Autodesk Fusion 360 part; units mm, degrees
note: some values were not read from the file. Set by a fixed rule: which sketch regions a step uses.
(part 2 of 2)
sketch "Sketch10" plane through (0, 25.4, 0) normal (0, 1, 0) x (-1, 0, 0)
  line L0 (-83.2873, -65.9474) -> (-83.2873, -59.1973)
  line L1 (-83.2873, -59.1973) -> (-104.0797, -59.1973)
  arc A0 (-123.262, -24.2329) -> (-104.0797, -59.1973) centre (-37.6354, -0.0001) ccw
  line L2 (-123.262, -24.2329) -> (-104.2867, -24.2329)
  line L3 (-104.2867, -24.2329) -> (-24.2324, -24.2327)
  line L4 (-24.2324, -24.2327) -> (-24.2324, -59.1973)
  line L5 (-24.2324, -59.1973) -> (-24.3061, -59.1973)
  line L6 (-24.3061, -59.1973) -> (-79.2873, -59.1973)
  line L7 (-79.2873, -59.1973) -> (-79.2873, -65.9474)
  line L8 (-79.2873, -65.9474) -> (-65.947, -65.9474)
  line L9 (-65.947, -65.9474) -> (-65.947, -107.6618)
  line L10 (-65.947, -107.6618) -> (-62.572, -107.6618)
  line L11 (-62.572, -107.6618) -> (-59.197, -107.6619)
  line L12 (-59.197, -107.6619) -> (-59.197, -107.6618)
  line L13 (-59.197, -107.6618) -> (65.9471, -107.6618)
  line L14 (65.9471, -107.6618) -> (65.9472, -104.2868)
  line L15 (65.9472, -104.2868) -> (65.9471, -65.9472)
  line L16 (65.9471, -65.9472) -> (100.9118, -65.9471)
  line L17 (100.9118, -65.9471) -> (100.9118, -104.2868)
  line L18 (100.9118, -104.2868) -> (107.6618, -104.2868)
  line L19 (107.6618, -104.2868) -> (107.6618, -23.7396)
  arc A1 (107.6618, -23.7396) -> (107.6618, 23.7395) centre (102.4721, -0.0001) ccw
  line L20 (107.6618, 23.7395) -> (100.9118, 23.7395)
  line L21 (100.9118, 23.7395) -> (100.9118, 17.4823)
  line L22 (100.9118, 17.4823) -> (104.2868, 17.4823)
  arc A2 (104.2868, -17.4824) -> (104.2868, 17.4823) centre (102.443, -0.0001) ccw
  line L23 (104.2868, -17.4824) -> (100.9118, -17.4824)
  line L24 (100.9118, -17.4824) -> (100.9118, -59.1971)
  line L25 (100.9118, -59.1971) -> (65.9471, -59.1972)
  line L26 (65.9471, -59.1972) -> (65.947, -17.4824)
  line L27 (65.947, -17.4824) -> (-17.4824, -17.4824)
  line L28 (-17.4824, -17.4824) -> (-17.4824, 17.4823)
  line L29 (-17.4824, 17.4823) -> (17.7085, 17.4823)
  arc A3 (17.7085, 17.4823) -> (65.7207, 17.4823) centre (41.7146, 20.7869) ccw
  line L30 (65.7207, 17.4823) -> (96.9118, 17.4823)
  line L31 (96.9118, 17.4823) -> (96.9118, 24.2323)
  line L32 (96.9118, 24.2323) -> (62.5606, 24.2322)
  line L33 (62.5606, 24.2322) -> (59.1856, 24.2322)
  line L34 (59.1856, 24.2322) -> (59.197, 20.8573)
  arc A4 (24.2323, 20.8573) -> (59.197, 20.8573) centre (41.7146, 20.7869) ccw
  line L35 (24.2323, 20.8573) -> (24.2323, 24.2322)
  line L36 (24.2323, 24.2322) -> (20.8573, 24.2323)
  line L37 (20.8573, 24.2323) -> (-17.4824, 24.2323)
  line L38 (-17.4824, 24.2323) -> (-17.4825, 100.9119)
  line L39 (-17.4825, 100.9119) -> (17.4821, 100.912)
  line L40 (17.4821, 100.912) -> (17.4821, 59.197)
  line L41 (17.4821, 59.197) -> (20.8571, 59.197)
  line L42 (20.8571, 59.197) -> (65.9469, 59.197)
  line L43 (65.9469, 59.197) -> (65.9469, 62.572)
  line L44 (65.9469, 62.572) -> (65.9468, 100.9119)
  line L45 (65.9468, 100.9119) -> (100.9118, 100.9119)
  line L46 (100.9118, 100.9119) -> (100.9118, 27.7395)
  line L47 (100.9118, 27.7395) -> (107.6618, 27.7395)
  line L48 (107.6618, 27.7395) -> (107.6618, 104.287)
  line L49 (107.6618, 104.287) -> (104.2868, 107.6568)
  line L50 (104.2868, 107.6568) -> (63.9876, 107.6568)
  arc A5 (63.9876, 107.6568) -> (-65.9473, 104.2867) centre (-0.0002, 68.2001) ccw
  line L51 (-65.9473, 104.2867) -> (-65.9473, 65.947)
  line L52 (-65.9473, 65.947) -> (-104.2867, 65.947)
  arc A6 (-104.2867, 65.947) -> (-107.6617, -63.1217) centre (-42.5552, -0.2457) ccw
  line L53 (-107.6617, -63.1217) -> (-107.6617, -104.2871)
  line L54 (-107.6617, -104.2871) -> (-104.2867, -104.2868)
  line L55 (-104.2867, -104.2868) -> (-100.9117, -104.287)
  line L56 (-100.9117, -104.287) -> (-100.9117, -65.9474)
  line L57 (-100.9117, -65.9474) -> (-83.2873, -65.9474)
  line L58 (-17.4824, -59.1973) -> (-17.4824, -24.2327)
  line L59 (-17.4824, -24.2327) -> (59.1971, -24.2325)
  line L60 (59.1971, -24.2325) -> (59.1971, -59.1972)
  line L61 (59.1971, -59.1972) -> (20.8574, -59.1972)
  line L62 (20.8574, -59.1972) -> (-17.4824, -59.1973)
  line L63 (-17.4824, -65.9474) -> (17.4824, -65.9473)
  line L64 (17.4824, -65.9473) -> (17.4824, -100.9118)
  line L65 (17.4824, -100.9118) -> (-59.197, -100.9118)
  line L66 (-59.197, -100.9118) -> (-59.197, -65.9474)
  line L67 (-59.197, -65.9474) -> (-17.4824, -65.9474)
  line L68 (-17.4824, -65.9474) -> (-17.4824, -65.9474)
  line L69 (24.2322, 104.287) -> (24.2321, 107.662)
  line L70 (24.2321, 107.662) -> (-56.8908, 107.6591)
  arc A7 (59.1968, 104.2869) -> (-56.8908, 107.6591) centre (-0.0002, 66.274) ccw
  line L71 (59.1968, 104.2869) -> (59.1969, 65.947)
  line L72 (59.1969, 65.947) -> (24.2322, 65.9469)
  line L73 (24.2322, 65.9469) -> (24.2322, 104.287)
  line L74 (24.2324, -100.9118) -> (24.2324, -65.9473)
  line L75 (24.2324, -65.9473) -> (59.1971, -65.9472)
  line L76 (59.1971, -65.9472) -> (59.1971, -100.9118)
  line L77 (59.1971, -100.9118) -> (24.2324, -100.9118)
  line L78 (-24.2324, 17.4823) -> (-24.2324, -17.4824)
  line L79 (-24.2324, -17.4824) -> (-100.9117, -17.4824)
  line L80 (-100.9117, -17.4824) -> (-100.9117, 17.4823)
  line L81 (-100.9117, 17.4823) -> (-24.2324, 17.4823)
  line L82 (-59.1972, 59.197) -> (-59.1973, 100.9118)
  line L83 (-59.1973, 100.9118) -> (-24.2324, 100.9119)
  line L84 (-24.2324, 100.9119) -> (-24.2324, 24.2323)
  line L85 (-24.2324, 24.2323) -> (-107.6617, 24.2323)
  line L86 (-107.6617, 24.2323) -> (-107.6616, -17.4824)
  line L87 (-107.6616, -17.4824) -> (-124.8909, -17.4824)
  arc A8 (-104.0798, 59.197) -> (-124.8909, -17.4824) centre (-37.6354, -0.0001) ccw
  line L88 (-104.0798, 59.197) -> (-59.1972, 59.197)
  line L89 (-17.4824, -59.1973) -> (-24.2324, -59.1973)
  line L90 (-24.2324, -59.1973) -> (-24.2324, -65.9474)
  line L91 (-24.2324, -65.9474) -> (-17.4824, -65.9474)
  line L92 (-17.4824, -65.9474) -> (-17.4824, -59.1973)
  dimension "d79" = 6.75
  measures "d79" distance of L58.start L4.end
extrude "Extrude11" add sketch "Sketch10" along normal blind 7 contours L67 L89 L90 L91 L92 bodies 2 1
sketch "Sketch11" plane through (0, 25.4, 0) normal (0, 1, 0) x (-1, 0, 0)
  line L0 (-24.2324, -65.9474) -> (-24.2324, -59.1973)
  line L1 (-24.2324, -59.1973) -> (-24.3061, -59.1973)
  line L2 (-24.3061, -59.1973) -> (-79.2873, -59.1973)
  line L3 (-79.2873, -59.1973) -> (-79.2873, -65.9474)
  line L4 (-79.2873, -65.9474) -> (-65.947, -65.9474)
  line L5 (-65.947, -65.9474) -> (-65.947, -107.6618)
  line L6 (-65.947, -107.6618) -> (-62.572, -107.6618)
  line L7 (-62.572, -107.6618) -> (-59.197, -107.6619)
  line L8 (-59.197, -107.6619) -> (-59.197, -107.6618)
  line L9 (-59.197, -107.6618) -> (65.9471, -107.6618)
  line L10 (65.9471, -107.6618) -> (65.9472, -104.2868)
  line L11 (65.9472, -104.2868) -> (65.9471, -65.9472)
  line L12 (65.9471, -65.9472) -> (100.9118, -65.9471)
  line L13 (100.9118, -65.9471) -> (100.9118, -104.2868)
  line L14 (100.9118, -104.2868) -> (107.6618, -104.2868)
  line L15 (107.6618, -104.2868) -> (107.6618, -23.7396)
  arc A0 (107.6618, -23.7396) -> (107.6618, 23.7395) centre (102.4721, -0.0001) ccw
  line L16 (107.6618, 23.7395) -> (100.9118, 23.7395)
  line L17 (100.9118, 23.7395) -> (100.9118, 17.4823)
  line L18 (100.9118, 17.4823) -> (104.2868, 17.4823)
  arc A1 (104.2868, -17.4824) -> (104.2868, 17.4823) centre (102.443, -0.0001) ccw
  line L19 (104.2868, -17.4824) -> (100.9118, -17.4824)
  line L20 (100.9118, -17.4824) -> (100.9118, -59.1971)
  line L21 (100.9118, -59.1971) -> (65.9471, -59.1972)
  line L22 (65.9471, -59.1972) -> (65.947, -17.4824)
  line L23 (65.947, -17.4824) -> (-17.4824, -17.4824)
  line L24 (-17.4824, -17.4824) -> (-17.4824, 17.4823)
  line L25 (-17.4824, 17.4823) -> (17.7085, 17.4823)
  arc A2 (17.7085, 17.4823) -> (65.7207, 17.4823) centre (41.7146, 20.7869) ccw
  line L26 (65.7207, 17.4823) -> (96.9118, 17.4823)
  line L27 (96.9118, 17.4823) -> (96.9118, 24.2323)
  line L28 (96.9118, 24.2323) -> (62.5606, 24.2322)
  line L29 (62.5606, 24.2322) -> (59.1856, 24.2322)
  line L30 (59.1856, 24.2322) -> (59.197, 20.8573)
  arc A3 (24.2323, 20.8573) -> (59.197, 20.8573) centre (41.7146, 20.7869) ccw
  line L31 (24.2323, 20.8573) -> (24.2323, 24.2322)
  line L32 (24.2323, 24.2322) -> (20.8573, 24.2323)
  line L33 (20.8573, 24.2323) -> (-17.4824, 24.2323)
  line L34 (-17.4824, 24.2323) -> (-17.4825, 100.9119)
  line L35 (-17.4825, 100.9119) -> (17.4821, 100.912)
  line L36 (17.4821, 100.912) -> (17.4821, 59.197)
  line L37 (17.4821, 59.197) -> (20.8571, 59.197)
  line L38 (20.8571, 59.197) -> (65.9469, 59.197)
  line L39 (65.9469, 59.197) -> (65.9469, 62.572)
  line L40 (65.9469, 62.572) -> (65.9468, 100.9119)
  line L41 (65.9468, 100.9119) -> (100.9118, 100.9119)
  line L42 (100.9118, 100.9119) -> (100.9118, 27.7395)
  line L43 (100.9118, 27.7395) -> (107.6618, 27.7395)
  line L44 (107.6618, 27.7395) -> (107.6618, 104.287)
  line L45 (107.6618, 104.287) -> (104.2868, 107.6568)
  line L46 (104.2868, 107.6568) -> (63.9876, 107.6568)
  arc A4 (63.9876, 107.6568) -> (-65.9473, 104.2867) centre (-0.0002, 68.2001) ccw
  line L47 (-65.9473, 104.2867) -> (-65.9473, 65.947)
  line L48 (-65.9473, 65.947) -> (-104.2867, 65.947)
  arc A5 (-104.2867, 65.947) -> (-107.6617, -63.1217) centre (-42.5552, -0.2457) ccw
  line L49 (-107.6617, -63.1217) -> (-107.6617, -104.2871)
  line L50 (-107.6617, -104.2871) -> (-104.2867, -104.2868)
  line L51 (-104.2867, -104.2868) -> (-100.9117, -104.287)
  line L52 (-100.9117, -104.287) -> (-100.9117, -65.9474)
  line L53 (-100.9117, -65.9474) -> (-83.2873, -65.9474)
  line L54 (-83.2873, -65.9474) -> (-83.2873, -59.1973)
  line L55 (-83.2873, -59.1973) -> (-104.0797, -59.1973)
  arc A6 (-123.262, -24.2329) -> (-104.0797, -59.1973) centre (-37.6354, -0.0001) ccw
  line L56 (-123.262, -24.2329) -> (-104.2867, -24.2329)
  line L57 (-104.2867, -24.2329) -> (-24.2324, -24.2327)
  line L58 (-24.2324, -24.2327) -> (-24.2324, -59.1973)
  line L59 (-24.2324, -59.1973) -> (-17.4824, -59.1973)
  line L60 (-17.4824, -59.1973) -> (-17.4824, -24.2327)
  line L61 (-17.4824, -24.2327) -> (59.1971, -24.2325)
  line L62 (59.1971, -24.2325) -> (59.1971, -59.1972)
  line L63 (59.1971, -59.1972) -> (20.8574, -59.1972)
  line L64 (20.8574, -59.1972) -> (-17.4824, -59.1973)
  line L65 (-17.4824, -59.1973) -> (-17.4824, -65.9474)
  line L66 (-17.4824, -65.9474) -> (17.4824, -65.9473)
  line L67 (17.4824, -65.9473) -> (17.4824, -100.9118)
  line L68 (17.4824, -100.9118) -> (-59.197, -100.9118)
  line L69 (-59.197, -100.9118) -> (-59.197, -65.9474)
  line L70 (-59.197, -65.9474) -> (-24.2324, -65.9474)
  line L71 (24.2322, 104.287) -> (24.2321, 107.662)
  line L72 (24.2321, 107.662) -> (-56.8908, 107.6591)
  arc A7 (59.1968, 104.2869) -> (-56.8908, 107.6591) centre (-0.0002, 66.274) ccw
  line L73 (59.1968, 104.2869) -> (59.1969, 65.947)
  line L74 (59.1969, 65.947) -> (24.2322, 65.9469)
  line L75 (24.2322, 65.9469) -> (24.2322, 104.287)
  line L76 (24.2324, -100.9118) -> (24.2324, -65.9473)
  line L77 (24.2324, -65.9473) -> (59.1971, -65.9472)
  line L78 (59.1971, -65.9472) -> (59.1971, -100.9118)
  line L79 (59.1971, -100.9118) -> (24.2324, -100.9118)
  line L80 (-24.2324, 17.4823) -> (-24.2324, -17.4824)
  line L81 (-24.2324, -17.4824) -> (-100.9117, -17.4824)
  line L82 (-100.9117, -17.4824) -> (-100.9117, 17.4823)
  line L83 (-100.9117, 17.4823) -> (-24.2324, 17.4823)
  line L84 (-59.1972, 59.197) -> (-59.1973, 100.9118)
  line L85 (-59.1973, 100.9118) -> (-24.2324, 100.9119)
  line L86 (-24.2324, 100.9119) -> (-24.2324, 24.2323)
  line L87 (-24.2324, 24.2323) -> (-107.6617, 24.2323)
  line L88 (-107.6617, 24.2323) -> (-107.6616, -17.4824)
  line L89 (-107.6616, -17.4824) -> (-124.8909, -17.4824)
  arc A8 (-104.0798, 59.197) -> (-124.8909, -17.4824) centre (-37.6354, -0.0001) ccw
  line L90 (-104.0798, 59.197) -> (-59.1972, 59.197)
  line L91 (-100.9117, -2.7929) -> (-107.6616, -2.7929)
  line L92 (-107.6616, -2.7929) -> (-107.6616, 1.2071)
  line L93 (-107.6616, 1.2071) -> (-100.9117, 1.2071)
  line L94 (-100.9117, 1.2071) -> (-100.9117, -2.7929)
  dimension "d82" = 4
  measures "d82" distance of L91.start L93.end
extrude "Extrude12" add sketch "Sketch11" along normal blind 7 separate body contours L82 L88 L91 L92 L93 L94 makes body 3
sketch "Sketch12" plane through (0, 25.4, 0) normal (0, 1, 0) x (-1, 0, 0)
  line L0 (-24.2324, -65.9474) -> (-24.2324, -59.1973)
  line L1 (-24.2324, -59.1973) -> (-24.3061, -59.1973)
  line L2 (-24.3061, -59.1973) -> (-79.2873, -59.1973)
  line L3 (-79.2873, -59.1973) -> (-79.2873, -65.9474)
  line L4 (-79.2873, -65.9474) -> (-65.947, -65.9474)
  line L5 (-65.947, -65.9474) -> (-65.947, -107.6618)
  line L6 (-65.947, -107.6618) -> (-62.572, -107.6618)
  line L7 (-62.572, -107.6618) -> (-59.197, -107.6619)
  line L8 (-59.197, -107.6619) -> (-59.197, -107.6618)
  line L9 (-59.197, -107.6618) -> (65.9471, -107.6618)
  line L10 (65.9471, -107.6618) -> (65.9472, -104.2868)
  line L11 (65.9472, -104.2868) -> (65.9471, -65.9472)
  line L12 (65.9471, -65.9472) -> (100.9118, -65.9471)
  line L13 (100.9118, -65.9471) -> (100.9118, -104.2868)
  line L14 (100.9118, -104.2868) -> (107.6618, -104.2868)
  line L15 (107.6618, -104.2868) -> (107.6618, -23.7396)
  arc A0 (107.6618, -23.7396) -> (107.6618, 23.7395) centre (102.4721, -0.0001) ccw
  line L16 (107.6618, 23.7395) -> (100.9118, 23.7395)
  line L17 (100.9118, 23.7395) -> (100.9118, 17.4823)
  line L18 (100.9118, 17.4823) -> (104.2868, 17.4823)
  arc A1 (104.2868, -17.4824) -> (104.2868, 17.4823) centre (102.443, -0.0001) ccw
  line L19 (104.2868, -17.4824) -> (100.9118, -17.4824)
  line L20 (100.9118, -17.4824) -> (100.9118, -59.1971)
  line L21 (100.9118, -59.1971) -> (65.9471, -59.1972)
  line L22 (65.9471, -59.1972) -> (65.947, -17.4824)
  line L23 (65.947, -17.4824) -> (-17.4824, -17.4824)
  line L24 (-17.4824, -17.4824) -> (-17.4824, 17.4823)
  line L25 (-17.4824, 17.4823) -> (17.7085, 17.4823)
  arc A2 (17.7085, 17.4823) -> (65.7207, 17.4823) centre (41.7146, 20.7869) ccw
  line L26 (65.7207, 17.4823) -> (96.9118, 17.4823)
  line L27 (96.9118, 17.4823) -> (96.9118, 24.2323)
  line L28 (96.9118, 24.2323) -> (62.5606, 24.2322)
  line L29 (62.5606, 24.2322) -> (59.1856, 24.2322)
  line L30 (59.1856, 24.2322) -> (59.197, 20.8573)
  arc A3 (24.2323, 20.8573) -> (59.197, 20.8573) centre (41.7146, 20.7869) ccw
  line L31 (24.2323, 20.8573) -> (24.2323, 24.2322)
  line L32 (24.2323, 24.2322) -> (20.8573, 24.2323)
  line L33 (20.8573, 24.2323) -> (-17.4824, 24.2323)
  line L34 (-17.4824, 24.2323) -> (-17.4825, 100.9119)
  line L35 (-17.4825, 100.9119) -> (17.4821, 100.912)
  line L36 (17.4821, 100.912) -> (17.4821, 59.197)
  line L37 (17.4821, 59.197) -> (20.8571, 59.197)
  line L38 (20.8571, 59.197) -> (65.9469, 59.197)
  line L39 (65.9469, 59.197) -> (65.9469, 62.572)
  line L40 (65.9469, 62.572) -> (65.9468, 100.9119)
  line L41 (65.9468, 100.9119) -> (100.9118, 100.9119)
  line L42 (100.9118, 100.9119) -> (100.9118, 27.7395)
  line L43 (100.9118, 27.7395) -> (107.6618, 27.7395)
  line L44 (107.6618, 27.7395) -> (107.6618, 104.287)
  line L45 (107.6618, 104.287) -> (104.2868, 107.6568)
  line L46 (104.2868, 107.6568) -> (63.9876, 107.6568)
  arc A4 (63.9876, 107.6568) -> (-65.9473, 104.2867) centre (-0.0002, 68.2001) ccw
  line L47 (-65.9473, 104.2867) -> (-65.9473, 65.947)
  line L48 (-65.9473, 65.947) -> (-104.2867, 65.947)
  arc A5 (-104.2867, 65.947) -> (-107.6617, -63.1217) centre (-42.5552, -0.2457) ccw
  line L49 (-107.6617, -63.1217) -> (-107.6617, -104.2871)
  line L50 (-107.6617, -104.2871) -> (-104.2867, -104.2868)
  line L51 (-104.2867, -104.2868) -> (-100.9117, -104.287)
  line L52 (-100.9117, -104.287) -> (-100.9117, -65.9474)
  line L53 (-100.9117, -65.9474) -> (-83.2873, -65.9474)
  line L54 (-83.2873, -65.9474) -> (-83.2873, -59.1973)
  line L55 (-83.2873, -59.1973) -> (-104.0797, -59.1973)
  arc A6 (-123.262, -24.2329) -> (-104.0797, -59.1973) centre (-37.6354, -0.0001) ccw
  line L56 (-123.262, -24.2329) -> (-104.2867, -24.2329)
  line L57 (-104.2867, -24.2329) -> (-24.2324, -24.2327)
  line L58 (-24.2324, -24.2327) -> (-24.2324, -59.1973)
  line L59 (-24.2324, -59.1973) -> (-17.4824, -59.1973)
  line L60 (-17.4824, -59.1973) -> (-17.4824, -24.2327)
  line L61 (-17.4824, -24.2327) -> (59.1971, -24.2325)
  line L62 (59.1971, -24.2325) -> (59.1971, -59.1972)
  line L63 (59.1971, -59.1972) -> (20.8574, -59.1972)
  line L64 (20.8574, -59.1972) -> (-17.4824, -59.1973)
  line L65 (-17.4824, -59.1973) -> (-17.4824, -65.9474)
  line L66 (-17.4824, -65.9474) -> (17.4824, -65.9473)
  line L67 (17.4824, -65.9473) -> (17.4824, -100.9118)
  line L68 (17.4824, -100.9118) -> (-59.197, -100.9118)
  line L69 (-59.197, -100.9118) -> (-59.197, -65.9474)
  line L70 (-59.197, -65.9474) -> (-24.2324, -65.9474)
  line L71 (24.2322, 104.287) -> (24.2321, 107.662)
  line L72 (24.2321, 107.662) -> (-56.8908, 107.6591)
  arc A7 (59.1968, 104.2869) -> (-56.8908, 107.6591) centre (-0.0002, 66.274) ccw
  line L73 (59.1968, 104.2869) -> (59.1969, 65.947)
  line L74 (59.1969, 65.947) -> (24.2322, 65.9469)
  line L75 (24.2322, 65.9469) -> (24.2322, 104.287)
  line L76 (24.2324, -100.9118) -> (24.2324, -65.9473)
  line L77 (24.2324, -65.9473) -> (59.1971, -65.9472)
  line L78 (59.1971, -65.9472) -> (59.1971, -100.9118)
  line L79 (59.1971, -100.9118) -> (24.2324, -100.9118)
  line L80 (-24.2324, 17.4823) -> (-24.2324, -17.4824)
  line L81 (-24.2324, -17.4824) -> (-100.9117, -17.4824)
  line L82 (-100.9117, -17.4824) -> (-100.9117, 17.4823)
  line L83 (-100.9117, 17.4823) -> (-24.2324, 17.4823)
  line L84 (-59.1972, 59.197) -> (-59.1973, 100.9118)
  line L85 (-59.1973, 100.9118) -> (-24.2324, 100.9119)
  line L86 (-24.2324, 100.9119) -> (-24.2324, 24.2323)
  line L87 (-24.2324, 24.2323) -> (-107.6617, 24.2323)
  line L88 (-107.6617, 24.2323) -> (-107.6616, -17.4824)
  line L89 (-107.6616, -17.4824) -> (-124.8909, -17.4824)
  arc A8 (-104.0798, 59.197) -> (-124.8909, -17.4824) centre (-37.6354, -0.0001) ccw
  line L90 (-104.0798, 59.197) -> (-59.1972, 59.197)
  line L91 (-110.8315, -24.2329) -> (-114.8315, -24.2329)
  line L92 (-114.8315, -24.2329) -> (-114.8315, -17.4824)
  line L93 (-114.8315, -17.4824) -> (-110.8315, -17.4824)
  line L94 (-110.8315, -17.4824) -> (-110.8315, -24.2329)
  dimension "d85" = 4
  dimension "d86" = 6.7505
  measures "d85" distance of L91.start L91.end
  measures "d86" distance of L91.start L93.end
extrude "Extrude13" add sketch "Sketch12" along normal blind 7 separate body contours L56 L89 L91 L92 L93 L94 makes body 4
sketch "Sketch13" plane through (0, 25.4, 0) normal (0, 1, 0) x (-1, 0, 0)
  line L0 (-24.2324, -65.9474) -> (-24.2324, -59.1973)
  line L1 (-24.2324, -59.1973) -> (-24.3061, -59.1973)
  line L2 (-24.3061, -59.1973) -> (-79.2873, -59.1973)
  line L3 (-79.2873, -59.1973) -> (-79.2873, -65.9474)
  line L4 (-79.2873, -65.9474) -> (-65.947, -65.9474)
  line L5 (-65.947, -65.9474) -> (-65.947, -107.6618)
  line L6 (-65.947, -107.6618) -> (-62.572, -107.6618)
  line L7 (-62.572, -107.6618) -> (-59.197, -107.6619)
  line L8 (-59.197, -107.6619) -> (-59.197, -107.6618)
  line L9 (-59.197, -107.6618) -> (65.9471, -107.6618)
  line L10 (65.9471, -107.6618) -> (65.9472, -104.2868)
  line L11 (65.9472, -104.2868) -> (65.9471, -65.9472)
  line L12 (65.9471, -65.9472) -> (100.9118, -65.9471)
  line L13 (100.9118, -65.9471) -> (100.9118, -104.2868)
  line L14 (100.9118, -104.2868) -> (107.6618, -104.2868)
  line L15 (107.6618, -104.2868) -> (107.6618, -23.7396)
  arc A0 (107.6618, -23.7396) -> (107.6618, 23.7395) centre (102.4721, -0.0001) ccw
  line L16 (107.6618, 23.7395) -> (100.9118, 23.7395)
  line L17 (100.9118, 23.7395) -> (100.9118, 17.4823)
  line L18 (100.9118, 17.4823) -> (104.2868, 17.4823)
  arc A1 (104.2868, -17.4824) -> (104.2868, 17.4823) centre (102.443, -0.0001) ccw
  line L19 (104.2868, -17.4824) -> (100.9118, -17.4824)
  line L20 (100.9118, -17.4824) -> (100.9118, -59.1971)
  line L21 (100.9118, -59.1971) -> (65.9471, -59.1972)
  line L22 (65.9471, -59.1972) -> (65.947, -17.4824)
  line L23 (65.947, -17.4824) -> (-17.4824, -17.4824)
  line L24 (-17.4824, -17.4824) -> (-17.4824, 17.4823)
  line L25 (-17.4824, 17.4823) -> (17.7085, 17.4823)
  arc A2 (17.7085, 17.4823) -> (65.7207, 17.4823) centre (41.7146, 20.7869) ccw
  line L26 (65.7207, 17.4823) -> (96.9118, 17.4823)
  line L27 (96.9118, 17.4823) -> (96.9118, 24.2323)
  line L28 (96.9118, 24.2323) -> (62.5606, 24.2322)
  line L29 (62.5606, 24.2322) -> (59.1856, 24.2322)
  line L30 (59.1856, 24.2322) -> (59.197, 20.8573)
  arc A3 (24.2323, 20.8573) -> (59.197, 20.8573) centre (41.7146, 20.7869) ccw
  line L31 (24.2323, 20.8573) -> (24.2323, 24.2322)
  line L32 (24.2323, 24.2322) -> (20.8573, 24.2323)
  line L33 (20.8573, 24.2323) -> (-17.4824, 24.2323)
  line L34 (-17.4824, 24.2323) -> (-17.4825, 100.9119)
  line L35 (-17.4825, 100.9119) -> (17.4821, 100.912)
  line L36 (17.4821, 100.912) -> (17.4821, 59.197)
  line L37 (17.4821, 59.197) -> (20.8571, 59.197)
  line L38 (20.8571, 59.197) -> (65.9469, 59.197)
  line L39 (65.9469, 59.197) -> (65.9469, 62.572)
  line L40 (65.9469, 62.572) -> (65.9468, 100.9119)
  line L41 (65.9468, 100.9119) -> (100.9118, 100.9119)
  line L42 (100.9118, 100.9119) -> (100.9118, 27.7395)
  line L43 (100.9118, 27.7395) -> (107.6618, 27.7395)
  line L44 (107.6618, 27.7395) -> (107.6618, 104.287)
  line L45 (107.6618, 104.287) -> (104.2868, 107.6568)
  line L46 (104.2868, 107.6568) -> (63.9876, 107.6568)
  arc A4 (63.9876, 107.6568) -> (-65.9473, 104.2867) centre (-0.0002, 68.2001) ccw
  line L47 (-65.9473, 104.2867) -> (-65.9473, 65.947)
  line L48 (-65.9473, 65.947) -> (-104.2867, 65.947)
  arc A5 (-104.2867, 65.947) -> (-107.6617, -63.1217) centre (-42.5552, -0.2457) ccw
  line L49 (-107.6617, -63.1217) -> (-107.6617, -104.2871)
  line L50 (-107.6617, -104.2871) -> (-104.2867, -104.2868)
  line L51 (-104.2867, -104.2868) -> (-100.9117, -104.287)
  line L52 (-100.9117, -104.287) -> (-100.9117, -65.9474)
  line L53 (-100.9117, -65.9474) -> (-83.2873, -65.9474)
  line L54 (-83.2873, -65.9474) -> (-83.2873, -59.1973)
  line L55 (-83.2873, -59.1973) -> (-104.0797, -59.1973)
  arc A6 (-123.262, -24.2329) -> (-104.0797, -59.1973) centre (-37.6354, -0.0001) ccw
  line L56 (-123.262, -24.2329) -> (-104.2867, -24.2329)
  line L57 (-104.2867, -24.2329) -> (-24.2324, -24.2327)
  line L58 (-24.2324, -24.2327) -> (-24.2324, -59.1973)
  line L59 (-24.2324, -59.1973) -> (-17.4824, -59.1973)
  line L60 (-17.4824, -59.1973) -> (-17.4824, -24.2327)
  line L61 (-17.4824, -24.2327) -> (59.1971, -24.2325)
  line L62 (59.1971, -24.2325) -> (59.1971, -59.1972)
  line L63 (59.1971, -59.1972) -> (20.8574, -59.1972)
  line L64 (20.8574, -59.1972) -> (-17.4824, -59.1973)
  line L65 (-17.4824, -59.1973) -> (-17.4824, -65.9474)
  line L66 (-17.4824, -65.9474) -> (17.4824, -65.9473)
  line L67 (17.4824, -65.9473) -> (17.4824, -100.9118)
  line L68 (17.4824, -100.9118) -> (-59.197, -100.9118)
  line L69 (-59.197, -100.9118) -> (-59.197, -65.9474)
  line L70 (-59.197, -65.9474) -> (-24.2324, -65.9474)
  line L71 (24.2322, 104.287) -> (24.2321, 107.662)
  line L72 (24.2321, 107.662) -> (-56.8908, 107.6591)
  arc A7 (59.1968, 104.2869) -> (-56.8908, 107.6591) centre (-0.0002, 66.274) ccw
  line L73 (59.1968, 104.2869) -> (59.1969, 65.947)
  line L74 (59.1969, 65.947) -> (24.2322, 65.9469)
  line L75 (24.2322, 65.9469) -> (24.2322, 104.287)
  line L76 (24.2324, -100.9118) -> (24.2324, -65.9473)
  line L77 (24.2324, -65.9473) -> (59.1971, -65.9472)
  line L78 (59.1971, -65.9472) -> (59.1971, -100.9118)
  line L79 (59.1971, -100.9118) -> (24.2324, -100.9118)
  line L80 (-24.2324, 17.4823) -> (-24.2324, -17.4824)
  line L81 (-24.2324, -17.4824) -> (-100.9117, -17.4824)
  line L82 (-100.9117, -17.4824) -> (-100.9117, 17.4823)
  line L83 (-100.9117, 17.4823) -> (-24.2324, 17.4823)
  line L84 (-59.1972, 59.197) -> (-59.1973, 100.9118)
  line L85 (-59.1973, 100.9118) -> (-24.2324, 100.9119)
  line L86 (-24.2324, 100.9119) -> (-24.2324, 24.2323)
  line L87 (-24.2324, 24.2323) -> (-107.6617, 24.2323)
  line L88 (-107.6617, 24.2323) -> (-107.6616, -17.4824)
  line L89 (-107.6616, -17.4824) -> (-124.8909, -17.4824)
  arc A8 (-104.0798, 59.197) -> (-124.8909, -17.4824) centre (-37.6354, -0.0001) ccw
  line L90 (-104.0798, 59.197) -> (-59.1972, 59.197)
  line L91 (-17.4824, 58.8722) -> (-24.2324, 58.8722)
  line L92 (-24.2324, 58.8722) -> (-24.2324, 65.6222)
  line L93 (-24.2324, 65.6222) -> (-17.4824, 65.6222)
  line L94 (-17.4824, 65.6222) -> (-17.4824, 58.8722)
  dimension "d89" = 6.75
  measures "d89" distance of L91.start L93.end
extrude "Extrude14" add sketch "Sketch13" along normal blind 7 separate body contours L34 L86 L91 L92 L93 L94 makes body 5
sketch "Sketch14" plane through (0, 32.4, 0) normal (0, 1, 0) x (-1, 0, 0)
  circle A0 centre (0, 0) radius 152.4
  line L0 (100.9118, -59.1971) -> (100.9118, -17.4824)
  line L1 (100.9118, -17.4824) -> (104.2868, -17.4824)
  arc A1 (104.2868, -17.4824) -> (104.2868, 17.4823) centre (102.443, -0.0001) ccw
  line L2 (104.2868, 17.4823) -> (100.9118, 17.4823)
  line L3 (100.9118, 17.4823) -> (100.9118, 23.7395)
  line L4 (100.9118, 23.7395) -> (107.6618, 23.7395)
  arc A2 (107.6618, -23.7396) -> (107.6618, 23.7395) centre (102.4721, -0.0001) ccw
  line L5 (107.6618, -23.7396) -> (107.6618, -104.2868)
  line L6 (107.6618, -104.2868) -> (100.9118, -104.2868)
  line L7 (100.9118, -104.2868) -> (100.9118, -65.9471)
  line L8 (100.9118, -65.9471) -> (65.9471, -65.9472)
  line L9 (65.9471, -65.9472) -> (65.9472, -104.2868)
  line L10 (65.9472, -104.2868) -> (65.9471, -107.6618)
  line L11 (65.9471, -107.6618) -> (-59.197, -107.6618)
  line L12 (-59.197, -107.6618) -> (-59.197, -107.6619)
  line L13 (-59.197, -107.6619) -> (-62.572, -107.6618)
  line L14 (-62.572, -107.6618) -> (-65.947, -107.6618)
  line L15 (-65.947, -107.6618) -> (-65.947, -65.9474)
  line L16 (-65.947, -65.9474) -> (-79.2873, -65.9474)
  line L17 (-79.2873, -65.9474) -> (-79.2873, -59.1973)
  line L18 (-79.2873, -59.1973) -> (-24.3061, -59.1973)
  line L19 (-24.3061, -59.1973) -> (-24.2324, -59.1973)
  line L20 (-24.2324, -59.1973) -> (-24.2324, -24.2327)
  line L21 (-24.2324, -24.2327) -> (-104.2867, -24.2329)
  line L22 (-104.2867, -24.2329) -> (-123.262, -24.2329)
  arc A3 (-123.262, -24.2329) -> (-104.0797, -59.1973) centre (-37.6354, -0.0001) ccw
  line L23 (-104.0797, -59.1973) -> (-83.2873, -59.1973)
  line L24 (-83.2873, -59.1973) -> (-83.2873, -65.9474)
  line L25 (-83.2873, -65.9474) -> (-100.9117, -65.9474)
  line L26 (-100.9117, -65.9474) -> (-100.9117, -104.287)
  line L27 (-100.9117, -104.287) -> (-104.2867, -104.2868)
  line L28 (-104.2867, -104.2868) -> (-107.6617, -104.2871)
  line L29 (-107.6617, -104.2871) -> (-107.6617, -63.1217)
  arc A4 (-104.2867, 65.947) -> (-107.6617, -63.1217) centre (-42.5552, -0.2457) ccw
  line L30 (-104.2867, 65.947) -> (-65.9473, 65.947)
  line L31 (-65.9473, 65.947) -> (-65.9473, 104.2867)
  arc A5 (63.9876, 107.6568) -> (-65.9473, 104.2867) centre (-0.0002, 68.2001) ccw
  line L32 (63.9876, 107.6568) -> (104.2868, 107.6568)
  line L33 (104.2868, 107.6568) -> (107.6618, 104.287)
  line L34 (107.6618, 104.287) -> (107.6618, 27.7395)
  line L35 (107.6618, 27.7395) -> (100.9118, 27.7395)
  line L36 (100.9118, 27.7395) -> (100.9118, 100.9119)
  line L37 (100.9118, 100.9119) -> (65.9468, 100.9119)
  line L38 (65.9468, 100.9119) -> (65.9469, 62.572)
  line L39 (65.9469, 62.572) -> (65.9469, 59.197)
  line L40 (65.9469, 59.197) -> (20.8571, 59.197)
  line L41 (20.8571, 59.197) -> (17.4821, 59.197)
  line L42 (17.4821, 59.197) -> (17.4821, 100.912)
  line L43 (17.4821, 100.912) -> (-17.4825, 100.9119)
  line L44 (-17.4825, 100.9119) -> (-17.4824, 24.2323)
  line L45 (-17.4824, 24.2323) -> (20.8573, 24.2323)
  line L46 (20.8573, 24.2323) -> (24.2323, 24.2322)
  line L47 (24.2323, 24.2322) -> (24.2323, 20.8573)
  arc A6 (24.2323, 20.8573) -> (59.197, 20.8573) centre (41.7146, 20.7869) ccw
  line L48 (59.197, 20.8573) -> (59.1856, 24.2322)
  line L49 (59.1856, 24.2322) -> (62.5606, 24.2322)
  line L50 (62.5606, 24.2322) -> (96.9118, 24.2323)
  line L51 (96.9118, 24.2323) -> (96.9118, 17.4823)
  line L52 (96.9118, 17.4823) -> (65.7207, 17.4823)
  arc A7 (17.7085, 17.4823) -> (65.7207, 17.4823) centre (41.7146, 20.7869) ccw
  line L53 (17.7085, 17.4823) -> (-17.4824, 17.4823)
  line L54 (-17.4824, 17.4823) -> (-17.4824, -17.4824)
  line L55 (-17.4824, -17.4824) -> (65.947, -17.4824)
  line L56 (65.947, -17.4824) -> (65.9471, -59.1972)
  line L57 (65.9471, -59.1972) -> (100.9118, -59.1971)
  line L58 (100.9118, 17.4823) -> (96.9118, 17.4823)
  line L59 (96.9118, 17.4823) -> (96.9118, 23.6253)
  line L60 (96.9118, 23.6253) -> (100.9118, 23.6253)
  line L61 (100.9118, 23.6253) -> (100.9118, 17.4823)
extrude "Extrude15" cut sketch "Sketch14" against normal blind 7 contours L3 L51 L58 L59 L60 L61 bodies 2
sketch "Sketch15" plane through (0, 32.4, 0) normal (0, 1, 0) x (-1, 0, 0)
  line L0 (96.9118, 23.6253) -> (100.9118, 23.6253)
  line L1 (100.9118, 23.6253) -> (100.9118, 23.7395)
  line L2 (100.9118, 23.7395) -> (107.6618, 23.7395)
  arc A0 (107.6618, -23.7396) -> (107.6618, 23.7395) centre (102.4721, -0.0001) ccw
  line L3 (107.6618, -23.7396) -> (107.6618, -104.2868)
  line L4 (107.6618, -104.2868) -> (100.9118, -104.2868)
  line L5 (100.9118, -104.2868) -> (100.9118, -65.9471)
  line L6 (100.9118, -65.9471) -> (65.9471, -65.9472)
  line L7 (65.9471, -65.9472) -> (65.9472, -104.2868)
  line L8 (65.9472, -104.2868) -> (65.9471, -107.6618)
  line L9 (65.9471, -107.6618) -> (-59.197, -107.6618)
  line L10 (-59.197, -107.6618) -> (-59.197, -107.6619)
  line L11 (-59.197, -107.6619) -> (-62.572, -107.6618)
  line L12 (-62.572, -107.6618) -> (-65.947, -107.6618)
  line L13 (-65.947, -107.6618) -> (-65.947, -65.9474)
  line L14 (-65.947, -65.9474) -> (-79.2873, -65.9474)
  line L15 (-79.2873, -65.9474) -> (-79.2873, -59.1973)
  line L16 (-79.2873, -59.1973) -> (-24.3061, -59.1973)
  line L17 (-24.3061, -59.1973) -> (-24.2324, -59.1973)
  line L18 (-24.2324, -59.1973) -> (-24.2324, -24.2327)
  line L19 (-24.2324, -24.2327) -> (-104.2867, -24.2329)
  line L20 (-104.2867, -24.2329) -> (-123.262, -24.2329)
  arc A1 (-123.262, -24.2329) -> (-104.0797, -59.1973) centre (-37.6354, -0.0001) ccw
  line L21 (-104.0797, -59.1973) -> (-83.2873, -59.1973)
  line L22 (-83.2873, -59.1973) -> (-83.2873, -65.9474)
  line L23 (-83.2873, -65.9474) -> (-100.9117, -65.9474)
  line L24 (-100.9117, -65.9474) -> (-100.9117, -104.287)
  line L25 (-100.9117, -104.287) -> (-104.2867, -104.2868)
  line L26 (-104.2867, -104.2868) -> (-107.6617, -104.2871)
  line L27 (-107.6617, -104.2871) -> (-107.6617, -63.1217)
  arc A2 (-104.2867, 65.947) -> (-107.6617, -63.1217) centre (-42.5552, -0.2457) ccw
  line L28 (-104.2867, 65.947) -> (-65.9473, 65.947)
  line L29 (-65.9473, 65.947) -> (-65.9473, 104.2867)
  arc A3 (63.9876, 107.6568) -> (-65.9473, 104.2867) centre (-0.0002, 68.2001) ccw
  line L30 (63.9876, 107.6568) -> (104.2868, 107.6568)
  line L31 (104.2868, 107.6568) -> (107.6618, 104.287)
  line L32 (107.6618, 104.287) -> (107.6618, 27.7395)
  line L33 (107.6618, 27.7395) -> (100.9118, 27.7395)
  line L34 (100.9118, 27.7395) -> (100.9118, 100.9119)
  line L35 (100.9118, 100.9119) -> (65.9468, 100.9119)
  line L36 (65.9468, 100.9119) -> (65.9469, 62.572)
  line L37 (65.9469, 62.572) -> (65.9469, 59.197)
  line L38 (65.9469, 59.197) -> (20.8571, 59.197)
  line L39 (20.8571, 59.197) -> (17.4821, 59.197)
  line L40 (17.4821, 59.197) -> (17.4821, 100.912)
  line L41 (17.4821, 100.912) -> (-17.4825, 100.9119)
  line L42 (-17.4825, 100.9119) -> (-17.4824, 24.2323)
  line L43 (-17.4824, 24.2323) -> (20.8573, 24.2323)
  line L44 (20.8573, 24.2323) -> (24.2323, 24.2322)
  line L45 (24.2323, 24.2322) -> (24.2323, 20.8573)
  arc A4 (24.2323, 20.8573) -> (59.197, 20.8573) centre (41.7146, 20.7869) ccw
  line L46 (59.197, 20.8573) -> (59.1856, 24.2322)
  line L47 (59.1856, 24.2322) -> (62.5606, 24.2322)
  line L48 (62.5606, 24.2322) -> (96.9118, 24.2323)
  line L49 (96.9118, 24.2323) -> (96.9118, 23.6253)
  circle A5 centre (0, 0) radius 152.4
  line L50 (107.6618, 27.7395) -> (100.9118, 27.7395)
  line L51 (100.9118, 27.7395) -> (100.9118, 23.6253)
  line L52 (100.9118, 23.6253) -> (107.6618, 23.6253)
  line L53 (107.6618, 23.6253) -> (107.6618, 27.7395)
extrude "Extrude16" cut sketch "Sketch15" against normal blind 7 contours L2 L33 L50 L51 L53 bodies 2
sketch "Sketch16" plane through (0, 32.4, 0) normal (0, 1, 0) x (-1, 0, 0)
  line L0 (100.9118, 23.6253) -> (100.9118, 100.9119)
  line L1 (100.9118, 100.9119) -> (65.9468, 100.9119)
  line L2 (65.9468, 100.9119) -> (65.9469, 62.572)
  line L3 (65.9469, 62.572) -> (65.9469, 59.197)
  line L4 (65.9469, 59.197) -> (20.8571, 59.197)
  line L5 (20.8571, 59.197) -> (17.4821, 59.197)
  line L6 (17.4821, 59.197) -> (17.4821, 100.912)
  line L7 (17.4821, 100.912) -> (-17.4825, 100.9119)
  line L8 (-17.4825, 100.9119) -> (-17.4824, 24.2323)
  line L9 (-17.4824, 24.2323) -> (20.8573, 24.2323)
  line L10 (20.8573, 24.2323) -> (24.2323, 24.2322)
  line L11 (24.2323, 24.2322) -> (24.2323, 20.8573)
  arc A0 (24.2323, 20.8573) -> (59.197, 20.8573) centre (41.7146, 20.7869) ccw
  line L12 (59.197, 20.8573) -> (59.1856, 24.2322)
  line L13 (59.1856, 24.2322) -> (62.5606, 24.2322)
  line L14 (62.5606, 24.2322) -> (96.9118, 24.2323)
  line L15 (96.9118, 24.2323) -> (96.9118, 23.6253)
  line L16 (96.9118, 23.6253) -> (100.9118, 23.6253)
  line L17 (96.9118, 23.6253) -> (100.9118, 23.6253)
  line L18 (100.9118, 23.6253) -> (100.9118, 24.2126)
  line L19 (100.9118, 24.2126) -> (96.9118, 24.2126)
  line L20 (96.9118, 24.2126) -> (96.9118, 23.6253)
extrude "Extrude17" cut sketch "Sketch16" against normal blind 7 contours L0 L15 L16 L17 L18 L19 L20 bodies 2
sketch "Sketch17" plane through (0, 25.4, 0) normal (0, 1, 0) x (-1, 0, 0)
  line L0 (107.6618, 23.7395) -> (107.6618, 104.287)
  line L1 (107.6618, 104.287) -> (104.2868, 107.6568)
  line L2 (104.2868, 107.6568) -> (63.9876, 107.6568)
  arc A0 (63.9876, 107.6568) -> (-65.9473, 104.2867) centre (-0.0002, 68.2001) ccw
  line L3 (-65.9473, 104.2867) -> (-65.9473, 65.947)
  line L4 (-65.9473, 65.947) -> (-104.2867, 65.947)
  arc A1 (-104.2867, 65.947) -> (-107.6617, -63.1217) centre (-42.5552, -0.2457) ccw
  line L5 (-107.6617, -63.1217) -> (-107.6617, -104.2871)
  line L6 (-107.6617, -104.2871) -> (-104.2867, -104.2868)
  line L7 (-104.2867, -104.2868) -> (-100.9117, -104.287)
  line L8 (-100.9117, -104.287) -> (-100.9117, -65.9474)
  line L9 (-100.9117, -65.9474) -> (-83.2873, -65.9474)
  line L10 (-83.2873, -65.9474) -> (-83.2873, -59.1973)
  line L11 (-83.2873, -59.1973) -> (-104.0797, -59.1973)
  arc A2 (-123.262, -24.2329) -> (-104.0797, -59.1973) centre (-37.6354, -0.0001) ccw
  line L12 (-123.262, -24.2329) -> (-104.2867, -24.2329)
  line L13 (-104.2867, -24.2329) -> (-24.2324, -24.2327)
  line L14 (-24.2324, -24.2327) -> (-24.2324, -59.1973)
  line L15 (-24.2324, -59.1973) -> (-17.4824, -59.1973)
  line L16 (-17.4824, -59.1973) -> (-17.4824, -24.2327)
  line L17 (-17.4824, -24.2327) -> (59.1971, -24.2325)
  line L18 (59.1971, -24.2325) -> (59.1971, -59.1972)
  line L19 (59.1971, -59.1972) -> (20.8574, -59.1972)
  line L20 (20.8574, -59.1972) -> (-17.4824, -59.1973)
  line L21 (-17.4824, -59.1973) -> (-17.4824, -65.9474)
  line L22 (-17.4824, -65.9474) -> (17.4824, -65.9473)
  line L23 (17.4824, -65.9473) -> (17.4824, -100.9118)
  line L24 (17.4824, -100.9118) -> (-59.197, -100.9118)
  line L25 (-59.197, -100.9118) -> (-59.197, -65.9474)
  line L26 (-59.197, -65.9474) -> (-24.2324, -65.9474)
  line L27 (-24.2324, -65.9474) -> (-24.2324, -59.1973)
  line L28 (-24.2324, -59.1973) -> (-24.3061, -59.1973)
  line L29 (-24.3061, -59.1973) -> (-79.2873, -59.1973)
  line L30 (-79.2873, -59.1973) -> (-79.2873, -65.9474)
  line L31 (-79.2873, -65.9474) -> (-65.947, -65.9474)
  line L32 (-65.947, -65.9474) -> (-65.947, -107.6618)
  line L33 (-65.947, -107.6618) -> (-62.572, -107.6618)
  line L34 (-62.572, -107.6618) -> (-59.197, -107.6619)
  line L35 (-59.197, -107.6619) -> (-59.197, -107.6618)
  line L36 (-59.197, -107.6618) -> (65.9471, -107.6618)
  line L37 (65.9471, -107.6618) -> (65.9472, -104.2868)
  line L38 (65.9472, -104.2868) -> (65.9471, -65.9472)
  line L39 (65.9471, -65.9472) -> (100.9118, -65.9471)
  line L40 (100.9118, -65.9471) -> (100.9118, -104.2868)
  line L41 (100.9118, -104.2868) -> (107.6618, -104.2868)
  line L42 (107.6618, -104.2868) -> (107.6618, -23.7396)
  arc A3 (107.6618, -23.7396) -> (107.6618, 23.7395) centre (102.4721, -0.0001) ccw
  line L43 (65.7207, 17.4823) -> (104.2868, 17.4823)
  arc A4 (104.2868, -17.4824) -> (104.2868, 17.4823) centre (102.443, -0.0001) ccw
  line L44 (104.2868, -17.4824) -> (100.9118, -17.4824)
  line L45 (100.9118, -17.4824) -> (100.9118, -59.1971)
  line L46 (100.9118, -59.1971) -> (65.9471, -59.1972)
  line L47 (65.9471, -59.1972) -> (65.947, -17.4824)
  line L48 (65.947, -17.4824) -> (-17.4824, -17.4824)
  line L49 (-17.4824, -17.4824) -> (-17.4824, 17.4823)
  line L50 (-17.4824, 17.4823) -> (17.7085, 17.4823)
  arc A5 (17.7085, 17.4823) -> (65.7207, 17.4823) centre (41.7146, 20.7869) ccw
  line L51 (100.9118, 100.9119) -> (100.9118, 24.2126)
  line L52 (100.9118, 24.2126) -> (96.9118, 24.2126)
  line L53 (96.9118, 24.2126) -> (96.9118, 24.2323)
  line L54 (96.9118, 24.2323) -> (62.5606, 24.2322)
  line L55 (62.5606, 24.2322) -> (59.1856, 24.2322)
  line L56 (59.1856, 24.2322) -> (59.197, 20.8573)
  arc A6 (24.2323, 20.8573) -> (59.197, 20.8573) centre (41.7146, 20.7869) ccw
  line L57 (24.2323, 20.8573) -> (24.2323, 24.2322)
  line L58 (24.2323, 24.2322) -> (20.8573, 24.2323)
  line L59 (20.8573, 24.2323) -> (-17.4824, 24.2323)
  line L60 (-17.4824, 24.2323) -> (-17.4825, 100.9119)
  line L61 (-17.4825, 100.9119) -> (17.4821, 100.912)
  line L62 (17.4821, 100.912) -> (17.4821, 59.197)
  line L63 (17.4821, 59.197) -> (20.8571, 59.197)
  line L64 (20.8571, 59.197) -> (65.9469, 59.197)
  line L65 (65.9469, 59.197) -> (65.9469, 62.572)
  line L66 (65.9469, 62.572) -> (65.9468, 100.9119)
  line L67 (65.9468, 100.9119) -> (100.9118, 100.9119)
  line L68 (24.2322, 104.287) -> (24.2321, 107.662)
  line L69 (24.2321, 107.662) -> (-56.8908, 107.6591)
  arc A7 (59.1968, 104.2869) -> (-56.8908, 107.6591) centre (-0.0002, 66.274) ccw
  line L70 (59.1968, 104.2869) -> (59.1969, 65.947)
  line L71 (59.1969, 65.947) -> (24.2322, 65.9469)
  line L72 (24.2322, 65.9469) -> (24.2322, 104.287)
  line L73 (24.2324, -100.9118) -> (24.2324, -65.9473)
  line L74 (24.2324, -65.9473) -> (59.1971, -65.9472)
  line L75 (59.1971, -65.9472) -> (59.1971, -100.9118)
  line L76 (59.1971, -100.9118) -> (24.2324, -100.9118)
  line L77 (-24.2324, 17.4823) -> (-24.2324, -17.4824)
  line L78 (-24.2324, -17.4824) -> (-100.9117, -17.4824)
  line L79 (-100.9117, -17.4824) -> (-100.9117, 17.4823)
  line L80 (-100.9117, 17.4823) -> (-24.2324, 17.4823)
  line L81 (-59.1972, 59.197) -> (-59.1973, 100.9118)
  line L82 (-59.1973, 100.9118) -> (-24.2324, 100.9119)
  line L83 (-24.2324, 100.9119) -> (-24.2324, 24.2323)
  line L84 (-24.2324, 24.2323) -> (-107.6617, 24.2323)
  line L85 (-107.6617, 24.2323) -> (-107.6616, -17.4824)
  line L86 (-107.6616, -17.4824) -> (-124.8909, -17.4824)
  arc A8 (-104.0798, 59.197) -> (-124.8909, -17.4824) centre (-37.6354, -0.0001) ccw
  line L87 (-104.0798, 59.197) -> (-59.1972, 59.197)
  line L88 (107.6618, -23.7396) -> (100.9118, -23.7396)
  line L89 (100.9118, -23.7396) -> (100.9118, -30.4896)
  line L90 (100.9118, -30.4896) -> (107.6618, -30.4896)
  line L91 (107.6618, -30.4896) -> (107.6618, -23.7396)
  dimension "d98" = 6.75
  measures "d98" distance of L42.end L90.end
extrude "Extrude18" add sketch "Sketch17" along normal blind 7 separate body contours L42 L45 L88 L89 L90 L91 makes body 6
hole "Hole1" at (104.3544, 25.4, -100.5884) direction (0, -1, 0) diameter 5.5 depth 30 tip angle 118 bodies 2
